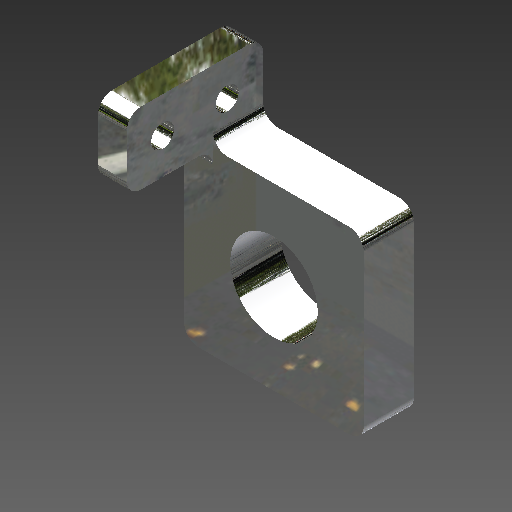
# Autodesk Inventor part: 3d_LM-Welding_Tooling - Fixed base
Saved by Autodesk Inventor 2018.3 (Build 223284000, 284)
## iProperties
Created: 2026-01-29
Part Number: 3d_LM-Welding_Tooling - Fixed base
Material: Aluminium 6061-T6
Document SubType Name: Modeling
Designer: aca6
Density: 2.7 g/cm^3
Appearance: N/A - Machined Aluminium
Manufacturer-1: {"Name": "Hanstar Technologies Co., Ltd", "PartNumber": "3d_Welding_Tooling - Fixed Block", "Link": ""}
Manufacturer-2: {"Name": "SHENZHEN JINYIHE PROTOTYPE TECHNOLOGIES CO., LTD", "PartNumber": "3d_Welding_Tooling - Fixed Block", "Link": ""}
Manufacturer-3: {"Name": "Shenzhen city Xavier Precision Co., Ltd.", "PartNumber": "3d_Welding_Tooling - Fixed Block", "Link": ""}
Manufacturer-4: {"Name": "", "PartNumber": "", "Link": ""}
Manufacturer-5: {"Name": "", "PartNumber": "", "Link": ""}
Provider-1: {"Name": "", "PartNumber": "", "Link": ""}
Provider-2: {"Name": "", "PartNumber": "", "Link": ""}
Provider-3: {"Name": "", "PartNumber": "", "Link": ""}
Provider-4: {"Name": "", "PartNumber": "", "Link": ""}
Provider-5: {"Name": "", "PartNumber": "", "Link": ""}
Author: aca6
Comments: DIN-ISO-2768-fH
Autodesk Inventor part; units mm, degrees
ref_plane "YZ Plane" through (0, 0, 0) normal (1, 0, 0) x (0, 1, 0)
ref_plane "XZ Plane" through (0, 0, 0) normal (0, 1, 0) x (-1, 0, 0)
ref_plane "XY Plane" through (0, 0, 0) normal (0, 0, 1) x (1, 0, 0)
sketch "Sketch1" plane through (0, 0, 0) normal (0, 0, 1) x (1, 0, 0)
  line L0 (-12.5, 22.5) -> (12.5, 22.5)
  line L1 (12.5, 22.5) -> (12.5, -22.5)
  line L2 (12.5, -22.5) -> (-12.5, -22.5)
  line L3 (-12.5, -22.5) -> (-12.5, 22.5)
  line L4 (0, 0) -> (0, 2.4254) construction
  line L5 (0, 0) -> (2.3845, 0) construction
  circle A0 centre (0, 0) radius 6.1
  dimension "d0" = 12.2
  dimension "d1" = 45
  dimension "d2" = 25
  constraints: 12 end point, 3 horizontal, 2 parallel, 2 vertical, 1 centre point, 1 coincident, 1 perpendicular, 4 other
  measures "d0" diameter of A0
  measures "d1" distance of L2.end L0.start
  measures "d2" distance of L0.start L0.end
extrude "Extrusion1" add sketch "Sketch1" along normal blind 7
sketch "Sketch2" plane through (12.5, -22.5, 0) normal (1, 0, 0) x (0, 0, -1)
  line L0 (-7, 45) -> (-7, 0) projected
  line L1 (0, 0) -> (-7, 0)
  line L2 (-7, 0) -> (-7, 10)
  line L3 (-7, 10) -> (0, 10)
  line L4 (0, 10) -> (0, 0)
  line L5 (0, 0) -> (0, 45) projected
  line L6 (-7, 45) -> (0, 45)
  line L7 (0, 45) -> (0, 35)
  line L8 (0, 35) -> (-7, 35)
  line L9 (-7, 35) -> (-7, 45)
  point P0 (0, 22.5)
  dimension "d5" = 10
  dimension "d6" = 10
  constraints: 16 end point, 4 parallel, 2 horizontal, 2 perpendicular, 2 point on line
  measures "d5" distance of L1.end L2.end
  measures "d6" distance of L6.end L7.end
extrude "Extrusion2" cut sketch "Sketch2" against normal through all contours L3 L4 L1 L0
sketch "Sketch3" plane through (12.5, 22.5, 7) normal (1, 0, 0) x (0, 0, -1)
  line L0 (7, 0) -> (0, 0) projected
  line L1 (0, -35) -> (0, 0) projected
  line L2 (7, 0) -> (0, 0)
  line L3 (0, 0) -> (0, -10)
  line L4 (0, -10) -> (7, -10)
  line L5 (7, -10) -> (7, 0)
  point P0 (7, -22.5)
  dimension "d9" = 10
  constraints: 8 end point, 2 parallel, 1 horizontal, 1 perpendicular, 1 point on line
  measures "d9" distance of L3.end L2.end
extrude "Extrusion3" cut sketch "Sketch3" against normal blind 16
sketch "Sketch4" plane through (0, 0, 7) normal (0, 0, 1) x (1, 0, 0)
  line L0 (-3.5, 22.5) -> (-12.5, 22.5) projected
  line L1 (-12.5, 22.5) -> (-12.5, -12.5) projected
  line L2 (-3.5, 22.5) -> (-12.5, 22.5)
  line L3 (-12.5, 22.5) -> (-12.5, 12.5)
  line L4 (-12.5, 12.5) -> (-3.5, 12.5)
  line L5 (-3.5, 12.5) -> (-3.5, 22.5)
  point P0 (0, 0)
  dimension "d12" = 10
  constraints: 8 end point, 2 parallel, 1 horizontal, 1 perpendicular, 1 point on line
  measures "d12" distance of L3.end L2.end
extrude "Extrusion4" add sketch "Sketch4" along normal blind 12
sketch "Sketch5" plane through (-3.5, 22.5, 7) normal (1, 0, 0) x (0, 0, -1)
  line L0 (-12, 0) -> (7, 0) projected
  line L1 (-12, -10) -> (-12, 0) projected
  point P0 (7, -22.5)
  point P1 (2, -5)
  point P2 (-7, -5)
  dimension "d15" = 5
  dimension "d17" = 9
  dimension "d30" = 5
  constraints: 1 horizontal alignment
  measures "d15" distance from line of L0 point (2, -5)
  measures "d17" distance of point (-7, -5) point (2, -5)
  measures "d30" distance from line of L1 point (-7, -5)
hole "Hole1" at (-3.5, 17.5, 5) at (-3.5, 17.5, 14) direction (-1, 0, 0) diameter 3.2 end through all
fillet "Fillet3" radius 2 3 edges at (12.5, -12.5, 3.5) (12.5, 12.5, 3.5) (-12.5, -12.5, 3.5)
sketch "Sketch6" plane through (-3.5, 22.5, 7) normal (1, 0, 0) x (0, 0, -1)
  circle A0 centre (2, -5) radius 1.6 projected
  circle A1 centre (-7, -5) radius 1.6 projected
  line L0 (-12, 0) -> (7, 0) projected
  line L1 (-12, -10) -> (-12, 0) projected
  line L2 (0, -10) -> (-12, -10) projected
  line L3 (7, -10) -> (0, -10) projected
  line L4 (7, 0) -> (7, -10) projected
  point P0 (7, -22.5)
extrude "Extrusion5" cut sketch "Sketch6" against normal blind 5
fillet "Fillet4" radius 2 5 edges at (-8.5, 12.5, 3.5) (-10.5, 12.5, 7) (-10.5, 12.5, 19) (-10.5, 22.5, 19) (-10.5, 22.5, 0)
body "Solid1"
